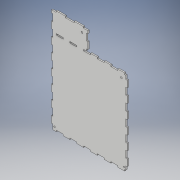
# Autodesk Inventor part: 8 zijplaat
Saved by Autodesk Inventor 2019 (Build 230136000, 136)
## iProperties
Created: 2021-01-22
Part Number: 8 zijplaat
Material: Generic
Document SubType Name: Sheet Metal
Designer: Stefan
Density: 1 g/cm^3
Sheet Metal Rule: Default_mm
Appearance: Default
Author: Stefan
Autodesk Inventor part; units mm, degrees
ref_plane "YZ Plane" through (0, 0, 0) normal (1, 0, 0) x (0, 1, 0)
ref_plane "XZ Plane" through (0, 0, 0) normal (0, 1, 0) x (-1, 0, 0)
ref_plane "XY Plane" through (0, 0, 0) normal (0, 0, 1) x (1, 0, 0)
sketch "Sketch1" plane through (0, 0, 0) normal (0, 0, 1) x (1, 0, 0)
  line L0 (-75, -90.5) -> (75, -90.5)
  line L1 (75, -90.5) -> (75, 90.5)
  line L2 (75, 90.5) -> (-75, 90.5)
  line L3 (-75, 90.5) -> (-75, -90.5)
  line L4 (-75, -90.5) -> (75, 90.5) construction
  line L5 (75, -90.5) -> (-75, 90.5) construction
  point P0 (0, 0)
  dimension "d0" = 150
  dimension "d1" = 181
  constraints: 12 end point, 2 midpoint, 2 parallel, 1 horizontal, 1 perpendicular
  measures "d0" distance of L2.end L1.end
  measures "d1" distance of L1.end L0.end
extrude "Extrusion1" add sketch "Sketch1" along normal blind 3
sketch "Sketch2" plane through (0, 0, 3) normal (0, 0, 1) x (1, 0, 0)
  line L0 (75, 90.5) -> (-75, 90.5) projected
  line L1 (-75, 90.5) -> (-67.5, 90.5)
  line L2 (-67.5, 90.5) -> (-67.5, 93.5)
  line L3 (-67.5, 93.5) -> (-75, 93.5)
  line L4 (-75, 93.5) -> (-75, 90.5)
  line L5 (67.5, 90.5) -> (75, 90.5)
  line L6 (75, 90.5) -> (75, 93.5)
  line L7 (75, 93.5) -> (67.5, 93.5)
  line L8 (67.5, 93.5) -> (67.5, 90.5)
  line L9 (-75, -93.5) -> (-67.5, -93.5)
  line L10 (-67.5, -93.5) -> (-67.5, -90.5)
  line L11 (-67.5, -90.5) -> (-75, -90.5)
  line L12 (-75, -90.5) -> (-75, -93.5)
  line L13 (67.5, -93.5) -> (75, -93.5)
  line L14 (75, -93.5) -> (75, -90.5)
  line L15 (75, -90.5) -> (67.5, -90.5)
  line L16 (67.5, -90.5) -> (67.5, -93.5)
  line L17 (-52.5, 90.5) -> (-37.5, 90.5)
  line L18 (-37.5, 90.5) -> (-37.5, 93.5)
  line L19 (-37.5, 93.5) -> (-52.5, 93.5)
  line L20 (-52.5, 93.5) -> (-52.5, 90.5)
  line L21 (-22.5, 90.5) -> (-7.5, 90.5)
  line L22 (-7.5, 93.5) -> (-22.5, 93.5)
  line L23 (-22.5, 93.5) -> (-22.5, 90.5)
  line L24 (-7.5, 90.5) -> (-7.5, 93.5)
  line L25 (7.5, 90.5) -> (22.5, 90.5)
  line L26 (22.5, 93.5) -> (7.5, 93.5)
  line L27 (7.5, 93.5) -> (7.5, 90.5)
  line L28 (22.5, 90.5) -> (22.5, 93.5)
  line L29 (37.5, 90.5) -> (52.5, 90.5)
  line L30 (52.5, 93.5) -> (37.5, 93.5)
  line L31 (37.5, 93.5) -> (37.5, 90.5)
  line L32 (52.5, 90.5) -> (52.5, 93.5)
  line L33 (-52.5, -93.5) -> (-37.5, -93.5)
  line L34 (-37.5, -90.5) -> (-52.5, -90.5)
  line L35 (-52.5, -90.5) -> (-52.5, -93.5)
  line L36 (-37.5, -93.5) -> (-37.5, -90.5)
  line L37 (-22.5, -93.5) -> (-7.5, -93.5)
  line L38 (-7.5, -90.5) -> (-22.5, -90.5)
  line L39 (-22.5, -90.5) -> (-22.5, -93.5)
  line L40 (-7.5, -93.5) -> (-7.5, -90.5)
  line L41 (7.5, -93.5) -> (22.5, -93.5)
  line L42 (22.5, -90.5) -> (7.5, -90.5)
  line L43 (7.5, -90.5) -> (7.5, -93.5)
  line L44 (22.5, -93.5) -> (22.5, -90.5)
  line L45 (37.5, -93.5) -> (52.5, -93.5)
  line L46 (52.5, -90.5) -> (37.5, -90.5)
  line L47 (37.5, -90.5) -> (37.5, -93.5)
  line L48 (52.5, -93.5) -> (52.5, -90.5)
  point P0 (0, 0)
  dimension "d4" = 7.5
  dimension "d5" = 3
  dimension "d8" = 142.5
  dimension "d11" = 184
  dimension "d14" = 15
  dimension "d15" = 3
  dimension "d16" = 15
  dimension "d19" = 30
  dimension "d22" = 184
  constraints: 96 end point, 4 horizontal, 4 parallel, 2 collinear, 2 perpendicular, 2 vertical, 1 point on line, 78 other
  measures "d4" distance of L3.end L2.end
  measures "d5" distance of L2.end L1.end
  measures "d8" distance of L2.end L6.end
  measures "d11" distance of L2.end L10.end
  measures "d14" distance of L19.end L18.end
  measures "d15" distance of L18.end L17.end
  measures "d16" distance between parallel lines of L20 L2
  measures "d19" distance of L17.end L21.end
  measures "d22" distance of L17.end L33.end
extrude "Extrusion2" add sketch "Sketch2" against normal blind 3
sketch "Sketch3" plane through (0, 0, 3) normal (0, 0, 1) x (1, 0, 0)
  line L0 (-75, 93.5) -> (-75, -93.5) projected
  line L1 (-75, 82.5) -> (-78, 82.5)
  line L2 (-78, 82.5) -> (-78, 67.5)
  line L3 (-78, 67.5) -> (-75, 67.5)
  line L4 (-75, 67.5) -> (-75, 82.5)
  line L5 (-75, 52.5) -> (-78, 52.5)
  line L6 (-78, 52.5) -> (-78, 37.5)
  line L7 (-78, 37.5) -> (-75, 37.5)
  line L8 (-75, 37.5) -> (-75, 52.5)
  line L9 (-75, 22.5) -> (-78, 22.5)
  line L10 (-78, 22.5) -> (-78, 7.5)
  line L11 (-78, 7.5) -> (-75, 7.5)
  line L12 (-75, 7.5) -> (-75, 22.5)
  line L13 (-75, -7.5) -> (-78, -7.5)
  line L14 (-78, -7.5) -> (-78, -22.5)
  line L15 (-78, -22.5) -> (-75, -22.5)
  line L16 (-75, -22.5) -> (-75, -7.5)
  line L17 (-75, -37.5) -> (-78, -37.5)
  line L18 (-78, -37.5) -> (-78, -52.5)
  line L19 (-78, -52.5) -> (-75, -52.5)
  line L20 (-75, -52.5) -> (-75, -37.5)
  line L21 (-75, -67.5) -> (-78, -67.5)
  line L22 (-78, -67.5) -> (-78, -82.5)
  line L23 (-78, -82.5) -> (-75, -82.5)
  line L24 (-75, -82.5) -> (-75, -67.5)
  line L25 (88, 82.5) -> (85, 82.5)
  line L26 (85, 82.5) -> (85, 67.5)
  line L27 (85, 67.5) -> (88, 67.5)
  line L28 (88, 67.5) -> (88, 82.5)
  line L29 (88, 52.5) -> (85, 52.5)
  line L30 (85, 52.5) -> (85, 37.5)
  line L31 (85, 37.5) -> (88, 37.5)
  line L32 (88, 37.5) -> (88, 52.5)
  line L33 (88, 22.5) -> (85, 22.5)
  line L34 (85, 22.5) -> (85, 7.5)
  line L35 (85, 7.5) -> (88, 7.5)
  line L36 (88, 7.5) -> (88, 22.5)
  line L37 (88, -7.5) -> (85, -7.5)
  line L38 (85, -7.5) -> (85, -22.5)
  line L39 (85, -22.5) -> (88, -22.5)
  line L40 (88, -22.5) -> (88, -7.5)
  line L41 (88, -37.5) -> (85, -37.5)
  line L42 (85, -37.5) -> (85, -52.5)
  line L43 (85, -52.5) -> (88, -52.5)
  line L44 (88, -52.5) -> (88, -37.5)
  line L45 (88, -67.5) -> (85, -67.5)
  line L46 (85, -67.5) -> (85, -82.5)
  line L47 (85, -82.5) -> (88, -82.5)
  line L48 (88, -82.5) -> (88, -67.5)
  point P0 (0, 0)
  dimension "d27" = 3
  dimension "d28" = 15
  dimension "d29" = 11
  dimension "d32" = 30
  dimension "d35" = 163
  constraints: 96 end point, 2 horizontal, 2 parallel, 1 collinear, 1 perpendicular, 1 point on line, 1 vertical, 87 other
  measures "d27" distance of L3.end L2.end
  measures "d28" distance of L2.end L1.end
  measures "d29" distance from line of L0.start L1
  measures "d32" distance of L1.start L5.start
  measures "d35" distance of L1.start L25.start
extrude "Extrusion3" add sketch "Sketch3" against normal blind 3
sketch "Sketch7" plane through (0, 0, 3) normal (0, 0, 1) x (1, 0, 0)
  line L0 (-75, 93.5) -> (-75, 82.5) projected
  line L1 (-75, 93.5) -> (-1.5, 93.5)
  line L2 (-78, 82.5) -> (-78, 97.5) construction
  line L3 (-78, 97.5) -> (-75, 97.5)
  line L4 (-75, 112.5) -> (-78, 112.5)
  line L5 (-78, 112.5) -> (-78, 97.5)
  line L6 (-75, 93.5) -> (-75, 97.5)
  line L7 (-75, 112.5) -> (-75, 127.5)
  line L8 (-75, 127.5) -> (-78, 127.5)
  line L9 (-78, 127.5) -> (-78, 133.5)
  line L10 (-78, 133.5) -> (1.5, 133.5)
  line L11 (1.5, 133.5) -> (1.5, 93.5) construction
  line L12 (1.5, 133.5) -> (1.5, 127.5)
  line L13 (1.5, 127.5) -> (-1.5, 127.5)
  line L14 (-1.5, 127.5) -> (-1.5, 112.5)
  line L15 (-1.5, 112.5) -> (1.5, 112.5)
  line L16 (1.5, 112.5) -> (1.5, 97.5)
  line L17 (1.5, 97.5) -> (-1.5, 97.5)
  line L18 (-1.5, 97.5) -> (-1.5, 93.5)
  point P0 (0, 0)
  dimension "d135" = 15
  dimension "d136" = 3
  dimension "d137" = 15
  dimension "d138" = 15
  dimension "d139" = 3
  dimension "d140" = 3
  dimension "d141" = 15
  dimension "d142" = 15
  dimension "d143" = 76.5
  dimension "d144" = 34
  dimension "d145" = 40
  dimension "d146" = 0
  constraints: 36 end point, 6 perpendicular, 6 point on line, 3 horizontal, 3 parallel, 2 vertical
  measures "d135" distance of L2.start L2.end
  measures "d136" distance of L4.end L4.start
  measures "d137" distance of L4.start L3.end
  measures "d138" distance of L4.start L7.end
  measures "d139" distance of L7.end L8.end
  measures "d140" distance of L12.end L13.end
  measures "d141" distance of L13.end L14.end
  measures "d142" distance of L15.end L16.end
  measures "d143" distance between parallel lines of L12 L0
  measures "d144" distance between parallel lines of L13 L1
  measures "d145" distance between parallel lines of L10 L1
  measures "d146" distance from line of L11.end L1
extrude "Extrusion6" add sketch "Sketch7" against normal blind 3
sketch "Sketch9" plane through (0, 0, 3) normal (0, 0, 1) x (1, 0, 0)
  line L0 (1.5, 133.5) -> (-78, 133.5) projected
  line L1 (-68.25, 133.5) -> (-48.25, 133.5)
  line L2 (-48.25, 133.5) -> (-48.25, 136.5)
  line L3 (-48.25, 136.5) -> (-68.25, 136.5)
  line L4 (-68.25, 136.5) -> (-68.25, 133.5)
  line L5 (-28.25, 133.5) -> (-8.25, 133.5)
  line L6 (-8.25, 133.5) -> (-8.25, 136.5)
  line L7 (-8.25, 136.5) -> (-28.25, 136.5)
  line L8 (-28.25, 136.5) -> (-28.25, 133.5)
  line L9 (-78, 133.5) -> (-78, 127.5) projected
  point P0 (0, 0)
  dimension "d164" = 20
  dimension "d165" = 3
  dimension "d168" = 40
  dimension "d173" = 9.75
  constraints: 16 end point, 2 horizontal, 2 parallel, 1 perpendicular, 1 point on line, 8 other
  measures "d164" distance of L3.end L2.end
  measures "d165" distance of L2.end L1.end
  measures "d168" distance of L1.start L5.start
  measures "d173" distance between parallel lines of L4 L9
extrude "Extrusion9" add sketch "Sketch9" against normal blind 3
sketch "Sketch10" plane through (0, 0, 3) normal (0, 0, 1) x (1, 0, 0)
  line L0 (67.5, 93.5) -> (75, 93.5) projected
  line L1 (67.5, 93.5) -> (82.5, 93.5)
  line L2 (82.5, 93.5) -> (82.5, 90.5)
  line L3 (82.5, 90.5) -> (67.5, 90.5)
  line L4 (67.5, 90.5) -> (67.5, 93.5)
  line L5 (67.5, -93.5) -> (67.5, -90.5) projected
  line L6 (67.5, -93.5) -> (82.5, -93.5)
  line L7 (82.5, -93.5) -> (82.5, -90.5)
  line L8 (82.5, -90.5) -> (67.5, -90.5)
  line L9 (67.5, -90.5) -> (67.5, -93.5)
  line L10 (85, 90.5) -> (85, -90.5)
  line L11 (85, -90.5) -> (75, -90.5)
  line L12 (75, 93.5) -> (75, -93.5) projected
  line L13 (75, -90.5) -> (75, 90.5)
  line L14 (75, 90.5) -> (85, 90.5)
  point P0 (0, 0)
  dimension "d176" = 15
  dimension "d177" = 3
  dimension "d178" = 10
  dimension "d179" = 7.5
  dimension "d180" = 184
  constraints: 24 end point, 5 parallel, 3 perpendicular, 2 horizontal, 2 midpoint, 1 point on line, 1 vertical
  measures "d176" distance of L2.end L3.end
  measures "d177" distance of L1.end L2.end
  measures "d178" distance between parallel lines of L10 L12
  measures "d179" distance between parallel lines of L7 L12
  measures "d180" distance between parallel lines of L8 L0
extrude "Extrusion10" add sketch "Sketch10" against normal blind 3
sketch "Sketch11" plane through (0, 0, 3) normal (0, 0, 1) x (1, 0, 0)
  circle A0 centre (-71.5, -86) radius 1.5
  circle A1 centre (81.5, -86) radius 1.5
  line L0 (88, -82.5) -> (88, -67.5) projected
  line L1 (67.5, -93.5) -> (82.5, -93.5) projected
  line L2 (-67.5, -93.5) -> (-75, -93.5) projected
  line L3 (-78, -67.5) -> (-78, -82.5) projected
  point P0 (0, 0)
  dimension "d183" = 3
  dimension "d184" = 3
  dimension "d185" = 6.5
  dimension "d186" = 7.5
  dimension "d187" = 7.5
  dimension "d188" = 6.5
  constraints: 2 centre point
  measures "d183" diameter of A0
  measures "d184" diameter of A1
  measures "d185" distance from line of L0 A1.centre
  measures "d186" distance from line of L1 A1.centre
  measures "d187" distance from line of L2 A0.centre
  measures "d188" distance from line of L3 A0.centre
extrude "Extrusion11" cut sketch "Sketch11" against normal blind 10
sketch "Sketch12" plane through (0, 0, 3) normal (0, 0, 1) x (1, 0, 0)
  circle A0 centre (75.5, 81) radius 2
  circle A1 centre (-11, 124) radius 2
  line L0 (-1.5, 112.5) -> (-1.5, 127.5) projected
  line L1 (1.5, 133.5) -> (-8.25, 133.5) projected
  line L2 (85, 82.5) -> (85, 90.5) projected
  line L3 (67.5, 90.5) -> (52.5, 90.5) projected
  point P0 (0, 0)
  dimension "d191" = 4
  dimension "d192" = 4
  dimension "d193" = 9.5
  dimension "d194" = 9.5
  dimension "d195" = 9.5
  dimension "d196" = 9.5
  constraints: 2 centre point
  measures "d191" diameter of A0
  measures "d192" diameter of A1
  measures "d193" distance from line of L0 A1.centre
  measures "d194" distance from line of L1 A1.centre
  measures "d195" distance from line of L2 A0.centre
  measures "d196" distance from line of L3 A0.centre
extrude "Extrusion12" cut sketch "Sketch12" against normal blind 10
equation "\"d187\" = d186"
equation "\"d188\" = d185"
equation "\"BendRadius\" = Thickness"
equation "\"BendReliefWidth\" = Thickness"
equation "\"BendReliefDepth\" = 0.5 * Thickness"
equation "\"CornerReliefSize\" = 4 * Thickness"
equation "\"MinimumRemnant\" = 2 * Thickness"
equation "\"TransitionRadius\" = BendRadius"
equation "\"JacobiRadiusSize\" = BendRadius"
equation "\"GapSize\" = Thickness"
equation "\"Thickness\" = 0.5"
body "Solid1"
